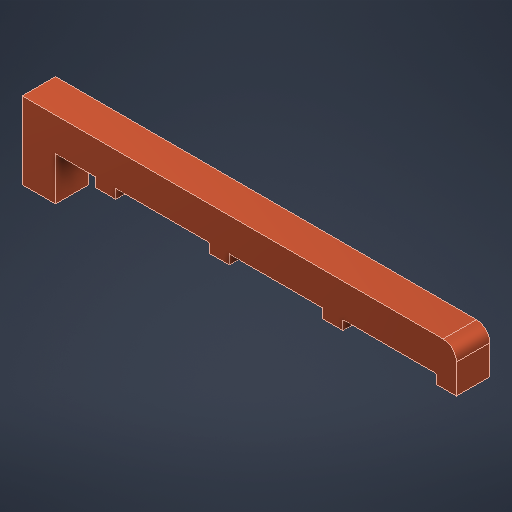
# Autodesk Inventor part: Bus_copper_top
Saved by Autodesk Inventor 2026.2 (Build 302298000, 298)
## iProperties
Created: 2025-12-09
Part Number: Bus_copper_top
Material: Медь
Document SubType Name: Modeling
Designer: EV-TECH
Density: 8.94 g/cm^3
Appearance: Медь — сатинированная
Author: EV-TECH
Autodesk Inventor part; units mm, degrees
ref_plane "YZ Plane" through (0, 0, 0) normal (1, 0, 0) x (0, 1, 0)
ref_plane "XZ Plane" through (0, 0, 0) normal (0, 1, 0) x (-1, 0, 0)
ref_plane "XY Plane" through (0, 0, 0) normal (0, 0, 1) x (1, 0, 0)
sketch "Эскиз1" plane through (0, 0, 0) normal (0, 1, 0) x (-1, 0, 0)
  line L0 (0, 0) -> (3, 0)
  line L1 (3, 0) -> (3, -5)
  line L2 (3, -5) -> (0, -5)
  line L3 (0, -5) -> (0, 0)
  line L4 (17, 0) -> (20, 0)
  line L5 (20, 0) -> (20, -5)
  line L6 (20, -5) -> (17, -5)
  line L7 (17, -5) -> (17, 0)
  line L8 (34, 0) -> (37, 0)
  line L9 (37, 0) -> (37, -5)
  line L10 (37, -5) -> (34, -5)
  line L11 (34, -5) -> (34, 0)
  line L12 (51, 0) -> (54, 0)
  line L13 (54, 0) -> (54, -5)
  line L14 (54, -5) -> (51, -5)
  line L15 (51, -5) -> (51, 0)
  dimension "d0" = 3
  dimension "d1" = 5
  dimension "d3" = 3
  dimension "d4" = 5
  dimension "d6" = 3
  dimension "d7" = 5
  dimension "d9" = 3
  dimension "d10" = 5
  constraints: 32 end point, 8 parallel, 4 horizontal, 4 perpendicular, 1 point on line
  measures "d0" distance of L1.end L2.end
  measures "d1" distance of L0.end L1.end
  measures "d3" distance of L5.end L6.end
  measures "d4" distance of L4.end L5.end
  measures "d6" distance of L9.end L10.end
  measures "d7" distance of L8.end L9.end
  measures "d9" distance of L13.end L14.end
  measures "d10" distance of L12.end L13.end
extrude "Выдавливание1" add sketch "Эскиз1" along normal blind 1.4
sketch "Эскиз2" plane through (0, 1.4, 0) normal (0, 1, 0) x (1, 0, 0)
  line L0 (0, 0) -> (-65, 0)
  line L1 (-65, 0) -> (-65, 5)
  line L2 (-65, 5) -> (0, 5)
  line L3 (0, 5) -> (0, 0)
  line L4 (-65, 0) -> (-60, 0)
  line L5 (-60, 5) -> (-65, 5)
  line L6 (-65, 5) -> (-65, 0)
  dimension "d14" = 65
  constraints: 14 end point, 3 parallel, 2 horizontal, 1 perpendicular
  measures "d14" distance of L1.end L2.end
extrude "Выдавливание2" add sketch "Эскиз2" along normal blind 5
fillet "Сопряжение1" radius 2 1 edges at (0, 6.4, -2.5)
sketch "Эскиз4" plane through (0, 1.4, 0) normal (0, -1, 0) x (1, 0, 0)
  line L0 (-65, 0) -> (-2, 0) projected
  line L1 (-65, 0) -> (-60, 0)
  line L2 (-60, 0) -> (-60, -5)
  line L3 (-60, -5) -> (-65, -5)
  line L4 (-65, -5) -> (-65, 0)
  point P0 (0, 0)
  dimension "d23" = 5
  dimension "d24" = 5
  constraints: 8 end point, 2 parallel, 1 horizontal, 1 perpendicular
  measures "d23" distance of L2.end L3.end
  measures "d24" distance of L3.end L0.start
extrude "Выдавливание3" add sketch "Эскиз4" along normal blind 6.5
